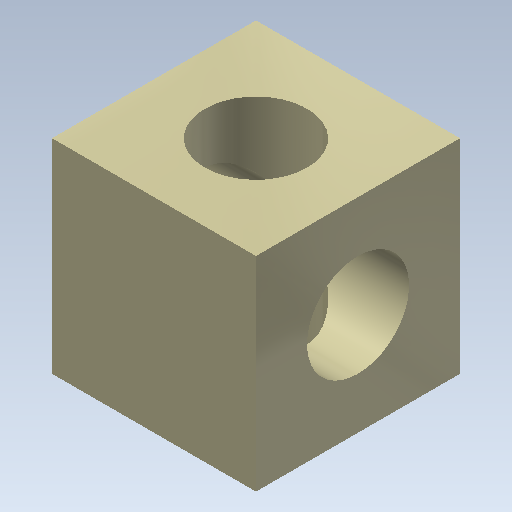
# Autodesk Inventor part: Connector
Saved by Autodesk Inventor 2021 Beta3 (Build 250176000, 176) ContinuousBuild 0
## iProperties
Created: 2014-03-03
Part Number: Connector
Material: Nylon 6/6
Document SubType Name: Modeling
Designer: John
Density: 1.13 g/cm^3
Appearance: Nylon 6
Mass: 1.59859 g
Surface Area: 11.8648 cm^2
Volume: 1.41468 cm^3
Author: John
Autodesk Inventor part; units mm, degrees
ref_plane "YZ Plane" through (0, 0, 0) normal (1, 0, 0) x (0, 1, 0)
ref_plane "XZ Plane" through (0, 0, 0) normal (0, 1, 0) x (-1, 0, 0)
ref_plane "XY Plane" through (0, 0, 0) normal (0, 0, 1) x (1, 0, 0)
sketch "Sketch1" plane through (0, 0, 0) normal (0, 0, 1) x (1, 0, 0)
  line L0 (-6.35, 6.35) -> (6.35, 6.35)
  line L1 (6.35, 6.35) -> (6.35, -6.35)
  line L2 (6.35, -6.35) -> (-6.35, -6.35)
  line L3 (-6.35, -6.35) -> (-6.35, 6.35)
  line L4 (-6.35, 6.35) -> (6.35, -6.35) construction
  line L5 (6.35, 6.35) -> (-6.35, -6.35) construction
  point P0 (0, 0)
  dimension "d0" = 12.7
  dimension "d1" = 12.7
  constraints: 12 end point, 2 midpoint, 2 parallel, 1 horizontal, 1 perpendicular
  measures "d0" distance of L1.end L2.end
  measures "d1" distance of L0.end L1.end
extrude "Extrusion1" add sketch "Sketch1" along normal blind 12.7
sketch "Sketch4" plane through (0, 0, 12.7) normal (0, 0, 1) x (1, 0, 0)
  point P0 (0, 0)
hole "Hole1" at (0, 0, 12.7) direction (0, 0, -1) diameter 6.35 end through all
sketch "Sketch5" plane through (6.35, -6.35, 0) normal (1, 0, 0) x (0, 0, -1)
  line L0 (-12.7, 12.7) -> (0, 0)
  point P0 (0, 6.35)
  point P1 (-6.35, 6.35)
  constraints: 2 end point, 1 midpoint
hole "Hole2" at (6.35, 0, 6.35) direction (-1, 0, 0) diameter 6.35 end through all
equation "\"d0\" = d1"
body "Solid1"
